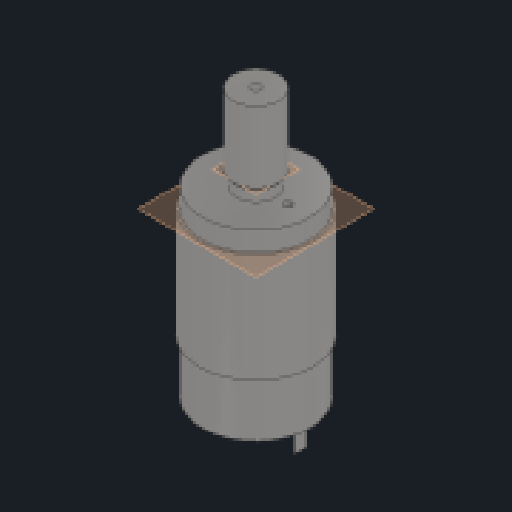
# Autodesk Inventor part: rs390
Saved by Autodesk Inventor 2023 (Build 270158000, 158)
## iProperties
Created: 2024-04-13
Part Number: rs390
Material: Steel, Mild
Document SubType Name: Modeling
Designer: szymo
Density: 7.85 g/cm^3
Appearance: Semi-Polished
Mass: 105 g
Surface Area: 71.7705 cm^2
Volume: 30.7913 cm^3
Author: szymo
Autodesk Inventor part; units mm, degrees
ref_plane "YZ Plane" through (0, 0, 0) normal (1, 0, 0) x (0, 1, 0)
ref_plane "XZ Plane" through (0, 0, 0) normal (0, 1, 0) x (-1, 0, 0)
ref_plane "XY Plane" through (0, 0, 0) normal (0, 0, 1) x (1, 0, 0)
sketch "Sketch1" plane through (0, 0, 0) normal (0, 1, 0) x (-1, 0, 0)
  circle A0 centre (0, 0) radius 13.7
  dimension "d0" = 27.4
  constraints: 1 centre point, 1 coincident
  measures "d0" diameter of A0
extrude "Extrusion1" add sketch "Sketch1" along normal blind 46.5
sketch "Sketch2" plane through (0, 46.5, 0) normal (0, 1, 0) x (1, 0, 0)
  circle A0 centre (0, 0) radius 13.7 projected
  circle A1 centre (0, 0) radius 5
  dimension "d3" = 10
  constraints: 1 centre point, 1 coincident
  measures "d3" diameter of A1
extrude "Extrusion2" add sketch "Sketch2" along normal blind 2.7 contours A1
sketch "Sketch3" plane through (0, 46.5, 0) normal (0, 1, 0) x (1, 0, 0)
  circle A0 centre (0, 0) radius 5 projected
  circle A1 centre (0, 0) radius 5 projected
  circle A2 centre (0, 0) radius 13.7 projected
  circle A3 centre (0, 0) radius 13.7 projected
  line L0 (-13.7, 0) -> (13.7, 0)
  point P0 (-8, 0)
  point P1 (8, 0)
  dimension "d6" = 16
  dimension "d7" = 5.7
  dimension "d8" = 5.7
  constraints: 2 end point, 2 point on circle, 2 point on line, 1 horizontal
  measures "d6" distance of point (-8, 0) point (8, 0)
  measures "d7" distance of L0.start point (-8, 0)
  measures "d8" distance of L0.end point (8, 0)
hole "Hole1" at (-8, 46.5, 0) at (8, 46.5, 0) direction (0, -1, 0) diameter 2.1129 depth 2.8 thread size "M2.6x0.45" class "6H" standard "ISO Metric profile"
ref_plane "Work Plane1" through (0, 41.5, 0) normal (0, 1, 0) x (1, 0, 0)
sketch "Sketch4" plane through (0, 41.5, 0) normal (0, 1, 0) x (1, 0, 0)
  circle A0 centre (0, 0) radius 14.375
  dimension "d17" = 28.75
  constraints: 1 centre point, 1 coincident
  measures "d17" diameter of A0
extrude "Extrusion3" add sketch "Sketch4" against normal blind 27.7
sketch "Sketch5" plane through (0, 0, 0) normal (0, -1, 0) x (1, 0, 0)
  circle A0 centre (0, 0) radius 5
  dimension "d20" = 10
  constraints: 1 centre point, 1 coincident
  measures "d20" diameter of A0
extrude "Extrusion4" add sketch "Sketch5" along normal blind 4
sketch "Sketch6" plane through (0, 0, 0) normal (0, -1, 0) x (1, 0, 0)
  circle A0 centre (0, 0) radius 5 projected
  circle A1 centre (0, 0) radius 5 projected
  circle A2 centre (0, 0) radius 13.7 projected
  circle A3 centre (0, 0) radius 13.7 projected
  line L0 (13.7, 0) -> (-13.7, 0)
  line L1 (-11.5, 1.5) -> (-12, 1.5)
  line L2 (-12, 1.5) -> (-12, -1.5)
  line L3 (-12, -1.5) -> (-11.5, -1.5)
  line L4 (-11.5, -1.5) -> (-11.5, 1.5)
  line L5 (11.5, 1.5) -> (11, 1.5)
  line L6 (11, 1.5) -> (11, -1.5)
  line L7 (11, -1.5) -> (11.5, -1.5)
  line L8 (11.5, -1.5) -> (11.5, 1.5)
  dimension "d23" = 22.5
  dimension "d24" = 0.5
  dimension "d25" = 0.5
  dimension "d26" = 11.5
  dimension "d27" = 11.5
  dimension "d28" = 3
  dimension "d29" = 3
  dimension "d30" = 1.5
  dimension "d31" = 1.5
  constraints: 18 end point, 4 horizontal, 4 parallel, 2 perpendicular, 2 point on circle, 2 point on line
  measures "d23" distance between parallel lines of L6 L4
  measures "d24" distance of L6.end L7.end
  measures "d25" distance between parallel lines of L4 L2
  measures "d26" distance from line of A2.centre L8
  measures "d27" distance from line of A0.centre L4
  measures "d28" distance between parallel lines of L3 L1
  measures "d29" distance of L7.end L5.start
  measures "d30" distance between parallel lines of L0 L7
  measures "d31" distance between parallel lines of L0 L5
extrude "Extrusion5" add sketch "Sketch6" along normal blind 6 contours L6 L5 L8 L0 | L0 L8 L7 L6 | L4 L3 L2 L0 | L0 L2 L1 L4
sketch "Sketch7" plane through (0, 49.2, 0) normal (0, 1, 0) x (1, 0, 0)
  circle A0 centre (0, 0) radius 1.1
  dimension "d34" = 2.2
  constraints: 1 centre point, 1 coincident
  measures "d34" diameter of A0
extrude "Extrusion6" add sketch "Sketch7" along normal blind 13.5
ref_plane "Work Plane2" through (0, 50.2, 0) normal (0, 1, 0) x (1, 0, 0)
sketch "Sketch9" plane through (0, 50.2, 0) normal (0, 1, 0) x (1, 0, 0)
  circle A0 centre (0, 0) radius 1.1 projected
  circle A1 centre (0, 0) radius 5.85
  dimension "d54" = 11.7
  constraints: 1 centre point, 1 coincident
  measures "d54" diameter of A1
extrude "Extrusion8" add sketch "Sketch9" along normal blind 18
equation "\"d7\" = d8"
equation "\"d26\" = d27"
equation "\"d30\" = d31"
equation "\"d41\" = d42"
body "Solid1"
